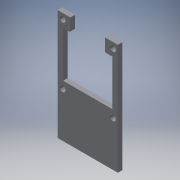
# Autodesk Inventor part: servotest
Saved by Autodesk Inventor 2018 (Build 220112000, 112)
## iProperties
Created: 2018-02-01
Part Number: servotest
Material: Generic
Document SubType Name: Modeling
Designer: Clevo
Density: 1 g/cm^3
Appearance: Default
Author: Clevo
Autodesk Inventor part; units mm, degrees
ref_plane "YZ Plane" through (0, 0, 0) normal (1, 0, 0) x (0, 1, 0)
ref_plane "XZ Plane" through (0, 0, 0) normal (0, 1, 0) x (-1, 0, 0)
ref_plane "XY Plane" through (0, 0, 0) normal (0, 0, 1) x (1, 0, 0)
sketch "Sketch1" plane through (0, 0, 0) normal (0, 1, 0) x (-1, 0, 0)
  line L0 (12.25, 22.5) -> (-12.25, 22.5)
  line L1 (-12.25, 22.5) -> (-12.25, -22.5)
  line L2 (-12.25, -22.5) -> (12.25, -22.5)
  line L3 (12.25, -22.5) -> (12.25, 22.5)
  point P0 (0, 0)
  point P1 (12.25, 0)
  point P2 (0, 22.5)
  dimension "d0" = 24.5
  dimension "d1" = 45
  constraints: 8 end point, 2 midpoint, 2 parallel, 1 horizontal, 1 horizontal alignment, 1 perpendicular, 1 vertical alignment
  measures "d0" distance of L2.end L1.end
  measures "d1" distance of L1.end L0.end
extrude "Extrusion1" add sketch "Sketch1" along normal blind 1.95
sketch "Sketch2" plane through (0, 1.95, 0) normal (0, 1, 0) x (1, 0, 0)
  line L0 (-10, 1.25) -> (10, 1.25)
  line L1 (10, 1.25) -> (10, -17.25)
  line L2 (10, -17.25) -> (-10, -17.25)
  line L3 (-10, -17.25) -> (-10, 1.25)
  line L4 (-12.25, -22.5) -> (12.25, -22.5) projected
  line L5 (12.25, -22.5) -> (12.25, 22.5) projected
  line L6 (12.25, 22.5) -> (-12.25, 22.5) projected
  line L7 (-12.25, 22.5) -> (-12.25, -22.5) projected
  line L8 (-7, -17.25) -> (7, -17.25)
  line L9 (7, -17.25) -> (7, -22.5)
  line L10 (7, -22.5) -> (-7, -22.5)
  line L11 (-7, -22.5) -> (-7, -17.25)
  line L12 (-12.25, -22.5) -> (12.25, -22.5) projected
  point P0 (0, 0)
  dimension "d4" = 2.25
  dimension "d5" = 20
  dimension "d6" = 2.25
  dimension "d7" = 5.25
  dimension "d8" = 5.25
  dimension "d9" = 14
  dimension "d10" = 5.25
  dimension "d11" = 18.5
  constraints: 16 end point, 4 parallel, 2 horizontal, 2 perpendicular, 1 collinear, 1 point on line
  measures "d4" distance between parallel lines of L7 L3
  measures "d5" distance of L0.start L0.end
  measures "d6" distance between parallel lines of L5 L1
  measures "d7" distance of L8.end L9.end
  measures "d8" distance between parallel lines of L7 L11
  measures "d9" distance between parallel lines of L9 L11
  measures "d10" distance between parallel lines of L5 L9
  measures "d11" distance of L0.end L1.end
extrude "Extrusion2" cut sketch "Sketch2" against normal up to surface (1.95 mm away) contours L0 L1 L2 L3 | L2 L9 L4 L11
sketch "Sketch3" plane through (0, 1.95, 0) normal (0, 1, 0) x (1, 0, 0)
  line L0 (-7, -22.5) -> (-7, -17.25) projected
  line L1 (-7, -17.25) -> (-10, -17.25) projected
  line L2 (-10, -17.25) -> (-10, 1.25) projected
  line L3 (-10, 1.25) -> (10, 1.25) projected
  line L4 (10, 1.25) -> (10, -17.25) projected
  line L5 (10, -17.25) -> (7, -17.25) projected
  line L6 (7, -17.25) -> (7, -22.5) projected
  line L7 (7, -22.5) -> (12.25, -22.5) projected
  line L8 (12.25, -22.5) -> (12.25, 22.5) projected
  line L9 (12.25, 22.5) -> (-12.25, 22.5) projected
  line L10 (-12.25, 22.5) -> (-12.25, -22.5) projected
  line L11 (-12.25, -22.5) -> (-7, -22.5) projected
  point P0 (0, 0)
  point P1 (-10.25, -20.305)
  point P2 (10.25, -20.305)
  dimension "d14" = 20.5
  dimension "d15" = 2
  dimension "d16" = 2.195
  dimension "d17" = 2
  constraints: 1 horizontal alignment
  measures "d14" distance of point (10.25, -20.305) point (-10.25, -20.305)
  measures "d15" distance from line of L8 point (10.25, -20.305)
  measures "d16" distance from line of L11 point (-10.25, -20.305)
  measures "d17" distance from line of L10 point (-10.25, -20.305)
hole "Hole1" at (-10.25, 1.95, 20.305) at (10.25, 1.95, 20.305) direction (0, -1, 0) diameter 2.4 end through all clearance for "Flat Head Machine Screw" size "M2" standard "Ansi Metric M Profile"
sketch "Sketch4" plane through (0, 1.95, 0) normal (0, 1, 0) x (1, 0, 0)
  circle A0 centre (-10.25, -20.305) radius 1.2 projected
  circle A1 centre (10.25, -20.305) radius 1.2 projected
  line L0 (-7, -22.5) -> (-7, -17.25) projected
  line L1 (-7, -17.25) -> (-10, -17.25) projected
  line L2 (-10, -17.25) -> (-10, 1.25) projected
  line L3 (-10, 1.25) -> (10, 1.25) projected
  line L4 (10, 1.25) -> (10, -17.25) projected
  line L5 (10, -17.25) -> (7, -17.25) projected
  line L6 (7, -17.25) -> (7, -22.5) projected
  line L7 (7, -22.5) -> (12.25, -22.5) projected
  line L8 (12.25, -22.5) -> (12.25, 22.5) projected
  line L9 (12.25, 22.5) -> (-12.25, 22.5) projected
  line L10 (-12.25, 22.5) -> (-12.25, -22.5) projected
  line L11 (-12.25, -22.5) -> (-7, -22.5) projected
  point P0 (0, 0)
  point P1 (-10.25, 4.15)
  point P2 (10.25, 4.15)
  dimension "d25" = 20.5
  dimension "d26" = 26.65
  dimension "d27" = 2
  dimension "d28" = 2
  constraints: 1 horizontal alignment
  measures "d25" distance of point (10.25, 4.15) point (-10.25, 4.15)
  measures "d26" distance from line of L11 point (-10.25, 4.15)
  measures "d27" distance from line of L10 point (-10.25, 4.15)
  measures "d28" distance from line of L8 point (10.25, 4.15)
hole "Hole2" at (-10.25, 1.95, -4.15) at (10.25, 1.95, -4.15) direction (0, -1, 0) diameter 2.4 end through all clearance for "Flat Head Machine Screw" size "M2" standard "Ansi Metric M Profile"
fillet "Fillet1" radius 0.5 2 edges at (7, 0.975, 17.25) (-7, 0.975, 17.25)
sketch "Sketch5" plane through (0, 1.95, 0) normal (0, 1, 0) x (1, 0, 0)
  circle A0 centre (-10.25, 4.15) radius 1.2 projected
  circle A1 centre (10.25, 4.15) radius 1.2 projected
  circle A2 centre (-10.25, -20.305) radius 1.2 projected
  circle A3 centre (10.25, -20.305) radius 1.2 projected
  arc A4 (-7, -17.75) -> (-7.5, -17.25) centre (-7.5, -17.75) ccw projected
  line L0 (-7.5, -17.25) -> (-10, -17.25) projected
  line L1 (-10, -17.25) -> (-10, 1.25) projected
  line L2 (-10, 1.25) -> (10, 1.25) projected
  line L3 (10, 1.25) -> (10, -17.25) projected
  line L4 (10, -17.25) -> (7.5, -17.25) projected
  arc A5 (7.5, -17.25) -> (7, -17.75) centre (7.5, -17.75) ccw projected
  line L5 (7, -17.75) -> (7, -22.5) projected
  line L6 (7, -22.5) -> (12.25, -22.5) projected
  line L7 (12.25, -22.5) -> (12.25, 22.5) projected
  line L8 (12.25, 22.5) -> (-12.25, 22.5) projected
  line L9 (-12.25, 22.5) -> (-12.25, -22.5) projected
  line L10 (-12.25, -22.5) -> (-7, -22.5) projected
  line L11 (-7, -22.5) -> (-7, -17.75) projected
  line L12 (-12.25, 22.5) -> (-12.25, -22.5) projected
  line L13 (12.25, -22.5) -> (12.25, 22.5) projected
  line L14 (-12.25, -22.5) -> (12.25, -22.5)
  line L15 (12.25, -22.5) -> (12.25, -4.5)
  line L16 (12.25, -4.5) -> (10, -4.5)
  line L17 (-12.25, -4.5) -> (-12.25, -22.5)
  line L18 (-10, -4.5) -> (-12.25, -4.5)
  line L19 (10, -4.5) -> (-10, -4.5)
  point P0 (0, 0)
  dimension "d37" = 18
  constraints: 12 end point, 4 parallel, 3 point on line, 1 horizontal, 1 perpendicular
  measures "d37" distance between parallel lines of L14 L16
extrude "Extrusion3" add sketch "Sketch5" along normal blind 5 contours L11 L10 L9 L18 L1 L0 A4 | A4 L0 L1 L19 L3 L4 A5 L5 L14 L11 | L5 A5 L4 L3 L16 L7 L6 | L18 L9 L8 L7 L16 L3 L2 L1
equation "\"d4\" = d6"
equation "\"d8\" = d10"
equation "\"d15\" = d17"
equation "\"d27\" = d28"
body "Solid1"
